Cyclone  Excenter (Autodesk Fusion 360 design; units mm, degrees)
Autodesk Fusion 360 part; units mm, degrees
other "Base Mesh Feature1"
ref_plane "WorkPlane1" through (0, 0, 0) normal (0, 1, 0) x (0, 0, 1)
sketch "Sketch1" plane through (0, 0, 0) normal (0, 1, 0) x (1, 0, 0)
  circle A0 centre (0, 0) radius 26
  circle A1 centre (0, 0) radius 28.5
  circle A2 centre (0, 0) radius 34.5
  dimension "d2" = 52
  dimension "d3" = 57
  dimension "d4" = 69
  constraint coincident A0.centre A1.centre
  constraint concentric A0 A2
  measures "d2" diameter of A0
  measures "d3" diameter of A1
  measures "d4" diameter of A2
extrude "Extrude1" add sketch "Sketch1" along normal blind 63 contours A1 makes body 1
extrude "Extrude2" add sketch "Sketch1" along normal blind 5 from surface at 58 contours A2 bodies 1
sketch "Sketch2" plane through (0, 0, 0) normal (0, 0, 1) x (1, 0, 0)
  line L0 (-7.5, 13) -> (-7.5, 6)
  line L1 (-7.5, 6) -> (7.5, 6)
  line L2 (7.5, 6) -> (7.5, 11)
  line L3 (7.5, 11) -> (-3.5, 11)
  line L4 (-3.5, 11) -> (-3.5, 13)
  line L5 (-3.5, 13) -> (-7.5, 13)
  constraint vertical L0
  constraint perpendicular L0 L1
  constraint perpendicular L1 L2
  constraint perpendicular L0 L3
  constraint perpendicular L1 L4
  constraint perpendicular L0 L5
extrude "Extrude3" add sketch "Sketch2" along normal blind 5.5 from surface at 26 bodies 1
fillet "Fillet1" radius 2 2 edges at (7.5, 6, 29.4977) (7.5, 11, 29.4977) on bodies 1
sketch "Sketch3" plane through (0, 63, 0) normal (0, 1, 0) x (-1, 0, 0)
  circle A0 centre (0, 0) radius 34.5
  circle A1 centre (0, 0) radius 26
  circle A2 centre (0, 0) radius 14.5
  circle A3 centre (0, 0) radius 11
  dimension "d15" = 29
  dimension "d16" = 22
  constraint coincident A0.centre A1.centre
  constraint concentric A2 A3
  measures "d15" diameter of A2
  measures "d16" diameter of A3
extrude "Extrude5" add sketch "Sketch3" against normal blind 5 contours A1 | A2 bodies 1
extrude "Extrude4" add sketch "Sketch3" along normal blind 35 contours A2 bodies 1
thread "Thread1" "ISO Metric profile 28.0 M28x2 6g" major diameter 27.822 minor diameter 25.5289 pitch 2 angle 60 modelled right hand crest width 0.2818 on face at (-14.4279, 86.3333, -1.4437) from (0, 68, 0) to (0, 98, 0) crest through (-13.911, 62.5, 0) on bodies 1
fillet "Fillet3" radius 25 1 edges at (-24.2405, 58, 9.402) on bodies 1
fillet "Fillet4" radius 5 1 edges at (12.9696, 63, 5.0304) on bodies 1
sketch "Sketch4" plane through (0, 58, 0) normal (0, -1, 0) x (1, 0, 0)
  circle A0 centre (0, 0) radius 28.5
  circle A1 centre (0, 0) radius 34.5
  circle A2 centre (0, 0) radius 28.7
  circle A3 centre (0, 0) radius 34.5
  dimension "d29" = 57.4
  dimension "d30" = 69
  constraint coincident A0.centre A1.centre
  measures "d29" diameter of A2
  measures "d30" diameter of A3
extrude "Extrude6" add sketch "Sketch4" along normal blind 8 separate body contours A1 A3 makes body 2
